Autodesk Inventor part; units mm, degrees
(part 2 of 2)
  line L408 (27.0607, 563.7766) -> (28.2267, 565.3313)
  line L409 (28.2267, 565.3313) -> (28.6752, 565.6004)
  line L410 (28.6752, 565.6004) -> (30.3197, 566.1984)
  line L411 (30.3197, 566.1984) -> (32.5622, 566.4077)
  line L412 (26.0441, 567.3645) -> (24.7883, 565.9891)
  line L413 (24.7883, 565.9891) -> (24.0109, 564.3746)
  line L414 (24.0109, 564.3746) -> (23.7119, 562.461)
  line L415 (23.7119, 562.461) -> (23.8614, 561.1753)
  line L416 (23.8614, 561.1753) -> (24.6089, 559.4113)
  line L417 (24.6089, 559.4113) -> (25.5657, 558.2452)
  line L418 (25.5657, 558.2452) -> (27.2401, 557.0791)
  line L419 (27.2401, 557.0791) -> (27.8979, 556.7801)
  line L420 (27.8979, 556.7801) -> (29.632, 556.1821)
  line L421 (29.632, 556.1821) -> (31.9941, 555.5542)
  line L422 (31.9941, 555.5542) -> (32.891, 555.3449)
  line L423 (32.891, 555.3449) -> (35.0737, 554.747)
  line L424 (35.0737, 554.747) -> (36.3893, 554.3284)
  line L425 (36.3893, 554.3284) -> (37.1966, 553.9995)
  line L426 (37.1966, 553.9995) -> (38.6317, 552.8932)
  line L427 (38.6317, 552.8932) -> (38.7812, 552.6839)
  line L428 (38.7812, 552.6839) -> (39.2895, 550.86)
  line L429 (39.2895, 550.86) -> (39.2895, 550.5311)
  line L430 (39.2895, 550.5311) -> (38.6018, 548.7372)
  line L431 (38.6018, 548.7372) -> (38.1832, 548.2289)
  line L432 (38.1832, 548.2289) -> (36.479, 547.2123)
  line L433 (36.479, 547.2123) -> (35.1933, 546.8236)
  line L434 (35.1933, 546.8236) -> (33.1601, 546.6442)
  line L435 (32.5622, 566.4077) -> (33.3993, 566.3778)
  line L436 (33.3993, 566.3778) -> (35.3727, 565.9891)
  line L437 (35.3727, 565.9891) -> (36.8677, 565.2117)
  line L438 (36.8677, 565.2117) -> (36.9873, 565.0921)
  line L439 (36.9873, 565.0921) -> (38.0636, 563.6271)
  line L440 (38.0636, 563.6271) -> (38.5719, 561.6537)
  line L441 (38.5719, 561.6537) -> (41.7114, 561.8929)
  line L442 (41.7114, 561.8929) -> (41.6815, 562.1321)
  line L443 (41.6815, 562.1321) -> (41.3227, 564.0756)
  line L444 (41.3227, 564.0756) -> (40.4855, 565.7798)
  line L445 (40.4855, 565.7798) -> (40.3061, 566.0489)
  line L446 (40.3061, 566.0489) -> (38.9905, 567.3944)
  line L447 (38.9905, 567.3944) -> (37.2863, 568.411)
  line L448 (37.2863, 568.411) -> (36.3594, 568.7399)
  line L449 (36.3594, 568.7399) -> (34.5056, 569.1585)
  line L450 (34.5056, 569.1585) -> (32.4127, 569.2781)
  line L451 (32.4127, 569.2781) -> (31.6652, 569.2482)
  line L452 (31.6652, 569.2482) -> (29.6918, 569.009)
  line L453 (29.6918, 569.009) -> (27.8979, 568.4409)
  line L454 (27.8979, 568.4409) -> (27.7484, 568.3811)
  line L455 (27.7484, 568.3811) -> (26.0441, 567.3645)
  line L456 (60.9367, 554.2985) -> (63.6276, 561.5341)
  line L457 (63.6276, 561.5341) -> (63.9565, 562.461)
  line L458 (63.9565, 562.461) -> (64.5246, 564.3447)
  line L459 (64.5246, 564.3447) -> (64.9731, 566.2582)
  line L460 (66.7969, 568.8595) -> (63.2688, 568.8595)
  line L461 (63.2688, 568.8595) -> (53.7907, 544.1327)
  line L462 (53.7907, 544.1327) -> (57.259, 544.1327)
  line L463 (57.259, 544.1327) -> (59.9799, 551.6075)
  line L464 (59.9799, 551.6075) -> (70.3251, 551.6075)
  line L465 (70.3251, 551.6075) -> (73.1954, 544.1327)
  line L466 (73.1954, 544.1327) -> (76.9029, 544.1327)
  line L467 (76.9029, 544.1327) -> (66.7969, 568.8595)
  line L468 (64.9731, 566.2582) -> (65.3319, 565.0921)
  line L469 (65.3319, 565.0921) -> (65.9299, 563.2683)
  line L470 (65.9299, 563.2683) -> (66.7072, 561.1454)
  line L471 (66.7072, 561.1454) -> (69.3085, 554.2985)
  line L472 (69.3085, 554.2985) -> (60.9367, 554.2985)
  line L473 (70.3251, 551.6075) -> (73.1954, 544.1327)
  line L474 (73.1954, 544.1327) -> (76.9029, 544.1327)
  line L475 (76.9029, 544.1327) -> (66.7969, 568.8595)
  line L476 (64.9731, 566.2582) -> (65.3319, 565.0921)
  line L477 (65.3319, 565.0921) -> (65.9299, 563.2683)
  line L478 (65.9299, 563.2683) -> (66.7072, 561.1454)
  line L479 (66.7072, 561.1454) -> (69.3085, 554.2985)
  line L480 (69.3085, 554.2985) -> (60.9367, 554.2985)
  line L481 (86.5903, 544.1327) -> (89.9391, 544.1327)
  line L482 (89.9391, 544.1327) -> (99.6264, 568.8595)
  line L483 (99.6264, 568.8595) -> (96.2777, 568.8595)
  line L484 (96.2777, 568.8595) -> (89.6102, 550.8899)
  line L485 (89.6102, 550.8899) -> (89.4906, 550.5909)
  line L486 (89.4906, 550.5909) -> (88.8627, 548.7372)
  line L487 (88.8627, 548.7372) -> (88.2647, 546.8535)
  line L488 (88.2647, 546.8535) -> (88.2049, 547.1226)
  line L489 (88.2049, 547.1226) -> (87.6368, 548.9465)
  line L490 (87.6368, 548.9465) -> (86.979, 550.8899)
  line L491 (86.979, 550.8899) -> (80.5506, 568.8595)
  line L492 (80.5506, 568.8595) -> (77.0225, 568.8595)
  line L493 (77.0225, 568.8595) -> (86.5903, 544.1327)
  line L494 (103.1247, 544.1327) -> (103.1247, 568.8595)
  line L495 (103.1247, 568.8595) -> (106.3837, 568.8595)
  line L496 (106.3837, 568.8595) -> (106.3837, 544.1327)
  line L497 (106.3837, 544.1327) -> (103.1247, 544.1327)
  line L498 (115.2937, 568.8595) -> (112.0048, 568.8595)
  line L499 (112.0048, 568.8595) -> (112.0048, 544.1327)
  line L500 (112.0048, 544.1327) -> (127.4628, 544.1327)
  line L501 (127.4628, 544.1327) -> (127.4628, 547.0628)
  line L502 (127.4628, 547.0628) -> (115.2937, 547.0628)
  line L503 (115.2937, 547.0628) -> (115.2937, 568.8595)
  line L504 (135.7449, 554.2985) -> (138.4657, 561.5341)
  line L505 (138.4657, 561.5341) -> (138.7946, 562.461)
  line L506 (138.7946, 562.461) -> (139.3627, 564.3447)
  line L507 (139.3627, 564.3447) -> (139.8112, 566.2582)
  line L508 (141.6351, 568.8595) -> (138.1069, 568.8595)
  line L509 (138.1069, 568.8595) -> (128.6288, 544.1327)
  line L510 (128.6288, 544.1327) -> (132.0972, 544.1327)
  line L511 (132.0972, 544.1327) -> (134.818, 551.6075)
  line L512 (134.818, 551.6075) -> (145.1333, 551.6075)
  line L513 (145.1333, 551.6075) -> (148.0335, 544.1327)
  line L514 (148.0335, 544.1327) -> (151.7411, 544.1327)
  line L515 (151.7411, 544.1327) -> (141.6351, 568.8595)
  line L516 (139.8112, 566.2582) -> (140.17, 565.0921)
  line L517 (140.17, 565.0921) -> (140.768, 563.2683)
  line L518 (140.768, 563.2683) -> (141.5454, 561.1454)
  line L519 (141.5454, 561.1454) -> (144.1466, 554.2985)
  line L520 (144.1466, 554.2985) -> (135.7449, 554.2985)
  line L521 (170.4581, 544.1327) -> (173.8068, 544.1327)
  line L522 (173.8068, 544.1327) -> (173.8068, 568.8595)
  line L523 (173.8068, 568.8595) -> (170.6674, 568.8595)
  line L524 (170.6674, 568.8595) -> (170.6674, 549.4548)
  line L525 (157.691, 568.8595) -> (154.3423, 568.8595)
  line L526 (154.3423, 568.8595) -> (154.3423, 544.1327)
  line L527 (154.3423, 544.1327) -> (157.4518, 544.1327)
  line L528 (157.4518, 544.1327) -> (157.4518, 563.5673)
  line L529 (170.6674, 549.4548) -> (157.691, 568.8595)
  line L530 (157.4518, 563.5673) -> (170.4581, 544.1327)
  line L531 (170.6674, 549.4548) -> (157.691, 568.8595)
  line L532 (157.4518, 563.5673) -> (170.4581, 544.1327)
  point P0 (0, 0)
  dimension "d0" = 300
  dimension "d1" = 400
  constraints: 1066 end point, 624 point on circle, 312 centre point, 2 midpoint, 2 parallel, 1 horizontal, 1 perpendicular
  measures "d0" distance of L1.end L2.end
  measures "d1" distance of L0.end L1.end
extrude "Extrusión1" add sketch "Boceto1" along normal blind 10 contours A283 A282 A281 A280 A279 A278 A277 A276 A275 A274 A273 A272 A271 A270 A269 A268 A267 A266 A265 A264 A263 A262 A261 A260 A259 A258 A257 A256 A255 A254 A253 A252 A251 A250 A249 A248 A247 A246 A245 A244 A243 A242 A241 A240 A239 A238 A237 A236 A235 A234 A233 A232 A231 A230 A229 A228 A227 A226 A225 A224 A223 A222 A221 A220 A219 A218 A217 A216 A215 A214 A213 A212 A211 A210 A209 A208 A207 A206 A205 A204 A203 A202 A201 A200 A199 A198 A197 A196 A195 A194 A193 A192 A191 A190 A189 A188 A187 A186 A185 A184 A183 A182 A181 A180 A179 A178 A177 A176 A175 A174 A173 A172 A171 A170 A169 A168 A167 A166 A165 A164 A163 A162 A161 A160 A159 A158 A157 A156 A155 A154 A153 A152 L11 L10 A151 A150 A149 A148 A147 A146 A145 A144 A143 A142 A141 A140 A139 A138 A137 A136 A135 A134 A133 A132 A131 A130 A129 A128 L9 L8 A127 A126 A125 A124 A123 A122 A121 A120 A119 A118 A117 A116 A115 A114 A113 A112 A111 A110 A109 A108 A107 A106 A105 A104 A103 A102 A101 A100 A99 A98 A97 A96 A95 A94 A93 A92 A91 A90 A89 A88 A87 A86 A85 A84 A83 A82 A81 A80 A79 A78 A77 A76 A75 A74 A73 A72 A71 A70 A69 A68 A67 A66 A65 A64 A63 A62 A61 A60 A59 A58 A57 A56 A55 A54 A53 A52 A51 A50 A49 A48 A47 A46 A45 A44 A43 A42 A41 A40 A39 A38 A37 A36 A35 A34 A33 A32 A31 A30 A29 A28 A27 A26 A25 A24 A23 A22 A21 A20 A19 A18 A17 A16 A15 A14 A13 A12 A11 A10 A9 A8 A7 A6 A5 A4 L7 L6 A3 A2 A1 A0 | L41 L40 L39 L38 L37 L36 L35 L34 L33 L32 L31 L30 L29 L28 L27 L26 L25 L24 L23 L22 L21 L20 L19 L18 L17 L16 L15 L14 L13 L12 | L82 L81 L80 L79 L78 L77 L76 L75 L74 L73 L72 L71 L70 L69 L68 L67 L66 L65 L64 L63 L62 L61 L60 L59 L58 L57 L56 L55 L54 L53 L52 L51 L50 L49 L48 L47 L46 L45 L44 L43 L42 | L94 L93 L92 L91 L90 L89 L88 L87 | L109 L107 L106 L105 L104 L108 L103 L102 L101 L100 | L132 L128 L127 L126 L125 L131 L130 L129 L118 L117 L116 L115 L114 L121 L120 L119 L113 L112 | L148 L147 L146 L145 L144 L143 L142 L141 L140 L139 L138 L137 | L161 L160 L159 L158 L157 L156 L155 L154 L153 L152 L151 L150 L149 | L173 L172 L171 L170 L169 L168 L167 L166 | L190 L189 L188 L187 L186 L185 L184 L183 | L205 L203 L202 L201 L200 L204 L199 L198 L197 L196 | L292 L291 L290 L289 L288 L287 L286 L285 L284 L281 L280 L279 L278 L277 L276 L221 L220 L219 L218 L217 L216 L215 L214 L213 L212 L211 L210 L209 L208 | L356 L355 L354 L353 L352 L345 L344 L343 L342 L329 L328 L327 L326 L325 L324 L323 L351 L350 L349 L348 L307 L306 L305 L304 L303 L302 L301 L300 L299 L298 L297 L296 L295 L294 L293 | L368 L367 L366 L365 L364 L363 L362 L361 L360 L359 L358 L357 | L434 L433 L432 L431 L430 L429 L428 L427 L426 L425 L424 L423 L422 L421 L420 L419 L418 L417 L416 L415 L414 L413 L412 L455 L454 L453 L452 L451 L450 L449 L448 L447 L446 L445 L444 L443 L442 L441 L440 L439 L438 L437 L436 L435 L411 L410 L409 L408 L407 L406 L405 L404 L403 L402 L401 L400 L399 L398 L397 L396 L395 L394 L393 L392 L391 L390 L389 L388 L387 L386 L385 L384 L383 L382 L381 L380 L379 L378 L377 L376 L375 L374 L373 L372 L371 L370 L369 | L467 L466 L465 L464 L463 L462 L461 L460 | L493 L492 L491 L490 L489 L488 L487 L486 L485 L484 L483 L482 L481 | L494 L495 L496 L497 | L503 L502 L501 L500 L499 L498 | L515 L514 L513 L512 L511 L510 L509 L508 | L530 L528 L527 L526 L525 L529 L524 L523 L522 L521
sketch "Boceto2" plane through (0, 0, 0) normal (0, -1, 0) x (1, 0, 0)
  line L0 (-247.8944, 657.766) -> (152.1056, 657.766)
  line L1 (152.1056, 657.766) -> (152.1056, 357.766)
  line L2 (152.1056, 357.766) -> (-247.8944, 357.766)
  line L3 (-247.8944, 357.766) -> (-247.8944, 657.766)
  point P0 (0, 0)
  dimension "d4" = 400
  dimension "d5" = 300
  constraints: 8 end point, 2 parallel, 1 horizontal, 1 perpendicular
  measures "d4" distance of L1.end L2.end
  measures "d5" distance of L0.end L1.end
extrude "Extrusión2" add sketch "Boceto2" along normal blind 100
